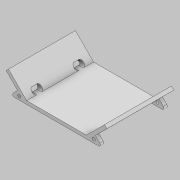
# Autodesk Inventor part: Soporte_electronica
Saved by Autodesk Inventor 2022.2 (Build 262287010, 287A)
## iProperties
Created: 2022-06-14
Part Number: Soporte_electronica
Material: Genérico
Document SubType Name: Modeling
Designer: Usuario
Density: 1 g/cm^3
Appearance: Valor por defecto
Author: Usuario
Autodesk Inventor part; units mm, degrees
ref_plane "YZ Plane" through (0, 0, 0) normal (1, 0, 0) x (0, 1, 0)
ref_plane "XZ Plane" through (0, 0, 0) normal (0, 1, 0) x (-1, 0, 0)
sketch "Boceto1" plane through (0, 0, 0) normal (0, 0, 1) x (1, 0, 0)
  line L0 (-52.7575, 20.0575) -> (-32.756, 0)
  line L1 (-32.756, 0) -> (0, 0)
  line L2 (-52.7575, 20.0575) -> (-50.2826, 22.5323)
  line L3 (-52.7575, 20.0575) -> (-49.2575, 20.0575) construction
  line L4 (-50.2826, 22.5323) -> (-31.3034, 3.5)
  line L5 (-31.3034, 3.5) -> (0, 3.5)
  line L6 (0, 0) -> (0, -9.9685) construction
  line L7 (52.7575, 20.0575) -> (32.756, 0)
  line L8 (32.756, 0) -> (0, 0)
  line L9 (52.7575, 20.0575) -> (50.2826, 22.5323)
  line L10 (50.2826, 22.5323) -> (31.3034, 3.5)
  line L11 (31.3034, 3.5) -> (0, 3.5)
  dimension "d0" = 45
  dimension "d1" = 134.92
  dimension "d2" = 3.5
  dimension "d3" = 3.5
  dimension "d4" = 28.326
  dimension "d5" = 32.756
  constraints: 24 end point, 4 symmetric about line, 3 horizontal, 1 equal length, 1 parallel, 1 vertical
  measures "d0" angle of L3 L2
  measures "d1" angle of L1 L0
  measures "d2" distance between parallel lines of L0 L4
  measures "d3" distance between parallel lines of L1 L5
  measures "d4" distance of L0.start L0.end
  measures "d5" distance of L0.end L1.end
extrude "Extrusión1" add sketch "Boceto1" along normal blind 70
sketch "Boceto2" plane through (0, 0, 70) normal (0, 0, 1) x (1, 0, 0)
  line L0 (-52.7575, 20.0575) -> (-32.756, 0) projected
  line L1 (-32.756, 0) -> (-48.756, 0)
  line L2 (-48.756, 0) -> (-40.7337, 8)
  line L3 (0, 0) -> (0, -7.1041) construction
  line L4 (52.7575, 20.0575) -> (32.756, 0)
  line L5 (32.756, 0) -> (48.756, 0)
  line L6 (48.756, 0) -> (40.7337, 8)
  point P0 (-47.756, 15.0419)
  dimension "d12" = 16
  constraints: 12 end point, 4 symmetric about line, 3 point on line, 1 horizontal, 1 perpendicular, 1 vertical
  measures "d12" distance of L1.end L0.end
extrude "Extrusión2" add sketch "Boceto2" against normal blind 3.5
ref_plane "Plano de trabajo1" through (0, 0, 35) normal (0, 0, 1) x (1, 0, 0)
mirror "Simetría1" about plane through (0, 0, 35) normal (0, 0, 1) of "Extrusión2"
sketch "Boceto3" plane through (0, 0, 70) normal (0, 0, 1) x (1, 0, 0)
  circle A0 centre (-39.0001, 3.8002) radius 1.5
  line L0 (-39.0001, 3.8002) -> (-37.7694, 5.0275) construction
  line L1 (-32.756, 0) -> (-40.7337, 8) projected
  line L2 (0, 0) -> (0, -3.5463) construction
  circle A1 centre (39.0001, 3.8002) radius 1.5
  dimension "d13" = 3
  dimension "d14" = 7.1
  dimension "d15" = 1.738
  constraints: 4 end point, 2 centre point, 1 perpendicular, 1 point on line, 1 symmetric about line, 1 vertical, 1 other
  measures "d13" diameter of A0
  measures "d14" distance of L0.end L1.start
  measures "d15" distance from line of L0.start L1
extrude "Extrusión3" cut sketch "Boceto3" against normal through all
fillet "Empalme1" radius 2 4 edges at (-48.756, 0, 68.25) (48.756, 0, 68.25) (48.756, 0, 1.75) (-48.756, 0, 1.75)
sketch "Boceto4" plane through (0, 0, 0) normal (1, 0, 0) x (0, 1, 0)
  line L0 (6, 62) -> (6, 52) construction
  line L1 (3.5, 59.5) -> (3.5, 54.5)
  line L2 (8.5, 54.5) -> (8.5, 59.5)
  arc A0 (8.5, 59.5) -> (3.5, 59.5) centre (6, 59.5) ccw
  arc A1 (3.5, 54.5) -> (8.5, 54.5) centre (6, 54.5) ccw
  line L3 (3.5, 70) -> (22.5323, 70) projected
  line L4 (3.5, 0) -> (3.5, 70) projected
  line L5 (0, 3.5) -> (0, 66.5) projected
  line L6 (0, 35) -> (-5.0365, 35) construction
  line L7 (3.5, 10.5) -> (3.5, 15.5)
  line L8 (8.5, 15.5) -> (8.5, 10.5)
  arc A2 (3.5, 10.5) -> (8.5, 10.5) centre (6, 10.5) ccw
  arc A3 (8.5, 15.5) -> (3.5, 15.5) centre (6, 15.5) ccw
  point P0 (0, 0)
  point P1 (6, 57)
  point P2 (3.5, 57)
  point P3 (3.5, 15.5)
  point P4 (3.5, 10.5)
  dimension "d19" = 10
  dimension "d20" = 5
  dimension "d21" = 8
  constraints: 14 end point, 11 point on circle, 6 symmetric about line, 4 centre point, 4 tangent, 3 midpoint, 3 point on line, 1 horizontal, 1 parallel, 1 vertical, 2 other
  measures "d19" distance of L0.start L0.end
  measures "d20" diameter of A1
  measures "d21" distance from line of L3 point (6, 62)
extrude "Extrusión4" cut sketch "Boceto4" along normal through all both and the other way through all
